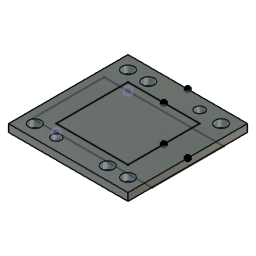
Membrane qui va marcher (Autodesk Fusion 360 archive; units mm, degrees)
design "Base flow plate"
Autodesk Fusion 360 part; units mm, degrees
sketch "Esquisse1" plane through (0, 0, 0) normal (0, 0, 1) x (1, 0, 0)
  line L0 (0, 0) -> (50, 0)
  line L1 (50, 0) -> (50, 50)
  line L2 (50, 50) -> (0, 50)
  line L3 (0, 50) -> (0, 0)
  dimension "d1" = 50
  dimension "d2" = 50
  constraint horizontal L0
  constraint vertical L1
  constraint horizontal L2
  constraint vertical L3
  constraint coincident L0.start L3.end
  measures "d1" distance of L1.end L2.end
  measures "d2" distance of L0.end L1.end
extrude "Extrusion1" add sketch "Esquisse1" along normal blind 3.175
sketch "Esquisse2" plane through (0, 0, 3.175) normal (0, 0, 1) x (-1, 0, 0)
  line L0 (0, -50) -> (0, 0)
  line L1 (0, 0) -> (-50, 0)
  line L2 (-50, 0) -> (-50, -50)
  line L3 (-50, -50) -> (0, -50)
  line L4 (-50, -50) -> (0, 0) construction
  circle A0 centre (-5.5, -44.5) radius 2.5
  circle A1 centre (-44.5, -44.5) radius 2.5
  circle A2 centre (-44.5, -5.5) radius 2.5
  circle A3 centre (-5.5, -5.5) radius 2.5
  line L5 (-44.5, -5.5) -> (-5.5, -44.5) construction
  line L6 (-5.5, -5.5) -> (-44.5, -44.5) construction
  point P0 (-47, -5.5)
  point P1 (-44.5, -3)
  dimension "d5" = 3
  dimension "d6" = 3
  dimension "d7" = 5
  constraint coincident L2.end L3.start
  constraint coincident L0.end L1.start
  constraint coincident A2.centre L5.start
  constraint coincident A0.centre L5.end
  constraint coincident A3.centre L6.start
  constraint coincident A1.centre L6.end
  constraint midpoint L5 L6
  constraint midpoint L4 L6
  constraint vertical A0.centre A3.centre
  constraint equal L5 L6
  constraint equal A0 A1
  constraint equal A1 A2
  constraint equal A2 A3
  constraint coincident A2 P0
  constraint coincident A2 P1
  constraint vertical A2.centre P1
  constraint horizontal A2.centre P0
  measures "d5" distance of L2 P0
  measures "d6" distance of L1 P1
  measures "d7" diameter of A1
extrude "Extrusion2" cut sketch "Esquisse2" against normal up to surface (3.175 mm away) contours A0 | A1 | A2 | A3
sketch "Esquisse3" plane through (0, 0, 3.175) normal (0, 0, 1) x (-1, 0, 0)
  circle A0 centre (-5.5, -5.5) radius 2.5
  circle A1 centre (-44.5, -5.5) radius 2.5
  circle A2 centre (-5.5, -44.5) radius 2.5
  circle A3 centre (-44.5, -44.5) radius 2.5
  line L0 (0, -50) -> (0, 0)
  line L1 (0, 0) -> (-50, 0)
  line L2 (-50, 0) -> (-50, -50)
  line L3 (-50, -50) -> (0, -50)
  line L4 (-50, -50) -> (0, 0) construction
  circle A4 centre (-35, -45) radius 2
  circle A5 centre (-15, -5) radius 2
  line L5 (-15, -5) -> (-35, -45) construction
  point P0 (-25, -25)
  point P1 (-35, -47)
  dimension "d10" = 4
  dimension "d11" = 10
  dimension "d12" = 3
  constraint coincident L2.end L3.start
  constraint coincident L0.end L1.start
  constraint coincident A5.centre L5.start
  constraint coincident A4.centre L5.end
  constraint midpoint L4 L5
  constraint equal A4 A5
  constraint midpoint L4 P0
  constraint coincident A4 P1
  constraint vertical A4.centre P1
  measures "d10" diameter of A5
  measures "d11" horizontal distance of A4.centre P0
  measures "d12" distance of L3 P1
extrude "Extrusion3" cut sketch "Esquisse3" against normal up to surface (3.175 mm away) contours A4 | A5
sketch "Esquisse4" plane through (0, 0, 3.175) normal (0, 0, 1) x (-1, 0, 0)
  circle A0 centre (-35, -45) radius 2
  circle A1 centre (-15, -5) radius 2
  circle A2 centre (-5.5, -5.5) radius 2.5
  circle A3 centre (-44.5, -5.5) radius 2.5
  circle A4 centre (-5.5, -44.5) radius 2.5
  circle A5 centre (-44.5, -44.5) radius 2.5
  line L0 (0, -50) -> (0, 0)
  line L1 (0, 0) -> (-50, 0)
  line L2 (-50, 0) -> (-50, -50)
  line L3 (-50, -50) -> (0, -50)
  line L4 (-10, -40) -> (-40, -40) construction
  line L5 (-40, -40) -> (-40, -10) construction
  line L6 (-40, -10) -> (-10, -10) construction
  line L7 (-10, -10) -> (-10, -40) construction
  line L8 (-10, -40) -> (-40, -10) construction
  line L9 (0, 0) -> (-50, -50) construction
  circle A6 centre (-14, -44.5) radius 2.5
  circle A7 centre (-36, -5.5) radius 2.5
  line L10 (-36, -5.5) -> (-14, -44.5) construction
  point P0 (-14, -42)
  dimension "d15" = 30
  dimension "d16" = 30
  dimension "d17" = 5
  dimension "d18" = 2
  dimension "d19" = 4
  constraint horizontal L4
  constraint vertical L5
  constraint horizontal L6
  constraint vertical L7
  constraint coincident L0.end L1.start
  constraint coincident L2.end L3.start
  constraint midpoint L8 L9
  constraint coincident A7.centre L10.start
  constraint coincident A6.centre L10.end
  constraint midpoint L9 L10
  constraint equal A6 A7
  constraint coincident A6 P0
  constraint vertical A6.centre P0
  measures "d15" distance of L5.end L6.end
  measures "d16" distance of L4.end L5.end
  measures "d17" diameter of A6
  measures "d18" distance of L4 P0
  measures "d19" horizontal distance of L4.start A6.centre
extrude "Extrusion4" cut sketch "Esquisse4" against normal up to surface (3.175 mm away) contours A6 | A7
sketch "Esquisse5" plane through (0, 0, 3.175) normal (0, 0, 1) x (-1, 0, 0)
  circle A0 centre (-14, -44.5) radius 2.5
  circle A1 centre (-36, -5.5) radius 2.5
  circle A2 centre (-35, -45) radius 2
  circle A3 centre (-15, -5) radius 2
  circle A4 centre (-5.5, -5.5) radius 2.5
  circle A5 centre (-44.5, -5.5) radius 2.5
  circle A6 centre (-5.5, -44.5) radius 2.5
  circle A7 centre (-44.5, -44.5) radius 2.5
  line L0 (0, -50) -> (0, 0)
  line L1 (0, 0) -> (-50, 0)
  line L2 (-50, 0) -> (-50, -50)
  line L3 (-50, -50) -> (0, -50)
  line L4 (-10, -40) -> (-40, -40)
  line L5 (-40, -40) -> (-40, -10)
  line L6 (-40, -10) -> (-10, -10)
  line L7 (-10, -10) -> (-10, -40)
  point P0 (-40, -25)
  point P1 (-50, -25)
  point P2 (-25, -40)
  point P3 (-25, -50)
  dimension "d22" = 30
  constraint horizontal L4
  constraint vertical L5
  constraint horizontal L6
  constraint vertical L7
  constraint midpoint L5 P0
  constraint midpoint L2 P1
  constraint midpoint L4 P2
  constraint midpoint L3 P3
  constraint vertical P2 P3
  constraint horizontal P0 P1
  constraint equal L4 L5
  measures "d22" distance of L4.start L6.end
sketch "Esquisse6" plane through (0, 0, 0) normal (0, 0, -1) x (1, 0, 0)
  circle A0 centre (14, -44.5) radius 2.5
  circle A1 centre (36, -5.5) radius 2.5
  circle A2 centre (35, -45) radius 2
  circle A3 centre (15, -5) radius 2
  circle A4 centre (5.5, -5.5) radius 2.5
  circle A5 centre (44.5, -5.5) radius 2.5
  circle A6 centre (5.5, -44.5) radius 2.5
  circle A7 centre (44.5, -44.5) radius 2.5
  line L0 (0, 0) -> (0, -50)
  line L1 (0, -50) -> (50, -50)
  line L2 (50, -50) -> (50, 0)
  line L3 (50, 0) -> (0, 0)
  line L4 (0, -10) -> (50, -10)
  line L5 (50, -10) -> (50, -40)
  line L6 (50, -40) -> (0, -40)
  line L7 (0, -40) -> (0, -10)
  point P0 (10, -40)
  point P1 (10, -10)
  constraint horizontal L4
  constraint vertical L5
  constraint horizontal L6
  constraint vertical L7
  constraint vertical L1.end L4.end
  constraint vertical L0.end L6.end
  constraint horizontal L6.end P0
  constraint horizontal L4.start P1
equation "d3 = 1 / 8 * 1 in"
